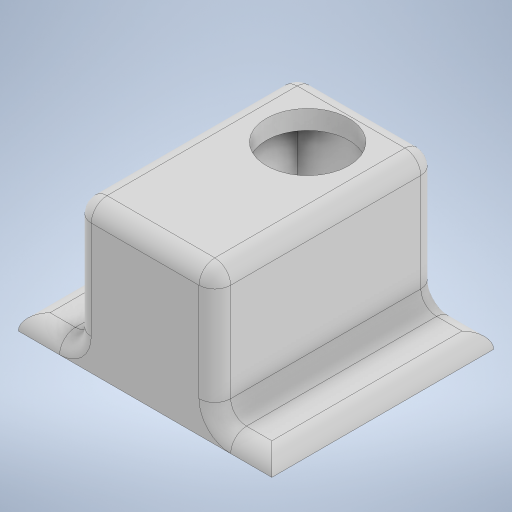
# Autodesk Inventor part: case_motor_inferior
Saved by Autodesk Inventor 2024 (Build 280153000, 153)
## iProperties
Created: 2024-10-14
Part Number: case_motor_inferior
Material: Genérico
Document SubType Name: Modeling
Designer: robof
Density: 1 g/cm^3
Appearance: Padrão
Author: robof
Autodesk Inventor part; units mm, degrees
ref_plane "YZ Plane" through (0, 0, 0) normal (1, 0, 0) x (0, 1, 0)
ref_plane "XZ Plane" through (0, 0, 0) normal (0, 1, 0) x (-1, 0, 0)
ref_plane "XY Plane" through (0, 0, 0) normal (0, 0, 1) x (1, 0, 0)
sketch "Esboço8" plane through (0, 0, 0) normal (0, 1, 0) x (-1, 0, 0)
  line L0 (0, 0) -> (-80, 0)
  line L1 (-80, 0) -> (-80, -70)
  line L2 (-80, -70) -> (0, -70)
  line L3 (0, -70) -> (0, 0)
  line L4 (0, 0) -> (-18, 0)
  line L5 (-80, -70) -> (-62, -70)
  line L6 (-18, 0) -> (-62, 0)
  line L7 (-62, 0) -> (-62, -70)
  line L8 (-62, -70) -> (-18, -70)
  line L9 (-18, -70) -> (-18, 0)
  dimension "d19" = 80
  dimension "d20" = 70
  dimension "d21" = 18
  dimension "d22" = 18
  constraints: 20 end point, 4 parallel, 2 horizontal, 2 perpendicular, 2 point on line
  measures "d19" distance of L2.end L1.end
  measures "d20" distance of L1.end L0.end
  measures "d21" distance of L0.start L4.end
  measures "d22" distance of L1.end L5.end
extrude "Extrusão6" add sketch "Esboço8" along normal blind 5 contours L3 L2 L9 L0 | L7 L2 L1 L0
sketch "Esboço9" plane through (0, 0, 0) normal (0, -1, 0) x (1, 0, 0)
  line L0 (0, 0) -> (18, 0) projected
  line L1 (62, -70) -> (62, 0) projected
  line L2 (18, 0) -> (62, 0)
  line L3 (62, 0) -> (62, -70)
  line L4 (62, -70) -> (18, -70)
  line L5 (18, -70) -> (18, 0)
  constraints: 8 end point, 2 parallel, 1 horizontal, 1 perpendicular
extrude "Extrusão7" add sketch "Esboço9" against normal blind 46
sketch "Esboço10" plane through (0, 0, 0) normal (0, -1, 0) x (1, 0, 0)
  line L0 (18, 0) -> (62, 0) projected
  line L1 (62, -70) -> (62, 0) projected
  line L2 (18, 0) -> (62, 0)
  line L3 (62, 0) -> (62, -70)
  line L4 (62, -70) -> (18, -70)
  line L5 (18, -70) -> (18, 0)
  line L6 (0, 0) -> (18, 0) projected
  line L7 (18, 0) -> (23, 0)
  line L8 (23, 0) -> (23, -5)
  line L9 (23, -5) -> (18, -5)
  line L10 (18, -5) -> (18, 0)
  line L11 (62, -70) -> (57, -70)
  line L12 (57, -70) -> (57, -65)
  line L13 (57, -65) -> (62, -65)
  line L14 (62, -65) -> (62, -70)
  line L15 (23, -5) -> (57, -5)
  line L16 (57, -5) -> (57, -65)
  line L17 (57, -65) -> (23, -65)
  line L18 (23, -65) -> (23, -5)
  dimension "d27" = 5
  dimension "d28" = 5
  dimension "d29" = 5
  dimension "d30" = 5
  constraints: 32 end point, 8 parallel, 4 horizontal, 4 perpendicular
  measures "d27" distance of L8.end L9.end
  measures "d28" distance of L7.end L8.end
  measures "d29" distance of L12.end L13.end
  measures "d30" distance of L11.end L12.end
extrude "Extrusão8" cut sketch "Esboço10" against normal blind 40 contours L15 L16 L17 L18
fillet "Arredondamento1" radius 5 16 edges at (62, 46, -35) (40, 46, 0) (18, 25.5, 0) (62, 25.5, 0) (62, 5, -35) (62, 25.5, -70) (80, 5, -35) (40, 46, -70) (18, 46, -35) (18, 25.5, -70) (18, 5, -35) (9, 5, -70) (9, 5, 0) (0, 5, -35) (71, 5, -70) (71, 5, 0)
sketch "Esboço11" plane through (0, 46, 0) normal (0, 1, 0) x (1, 0, 0)
  line L0 (23, 65) -> (23, 5) projected
  line L1 (57, 5) -> (57, 65) projected
  line L2 (23, 5) -> (57, 5)
  line L3 (57, 5) -> (57, 65)
  line L4 (57, 65) -> (23, 65)
  line L5 (23, 65) -> (23, 5)
  line L6 (40, 65) -> (40, 51.3)
  circle A0 centre (40, 51.3) radius 13
  point P0 (0, 0)
  dimension "d34" = 13.7
  dimension "d35" = 26
  constraints: 10 end point, 2 parallel, 1 centre point, 1 coincident, 1 horizontal, 1 midpoint, 1 perpendicular, 1 vertical
  measures "d34" distance of L6.start L6.end
  measures "d35" diameter of A0
extrude "Extrusão9" cut sketch "Esboço11" against normal blind 10 contours A0
